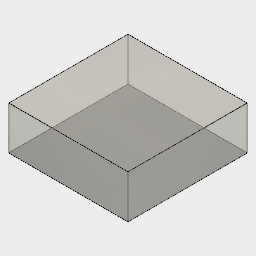
Poseidon thrust frame motor mount blocks (Autodesk Fusion 360 design; units mm, degrees)
Autodesk Fusion 360 part; units mm, degrees
sketch "Sketch1" plane through (0, 0, 0) normal (0, 1, 0) x (1, 0, 0)
  line L0 (0, 0) -> (34.925, 0)
  line L1 (34.925, 0) -> (34.925, 34.925)
  line L2 (34.925, 34.925) -> (0, 34.925)
  line L3 (0, 34.925) -> (0, 0)
  line L4 (0, 0) -> (34.925, 0)
  line L5 (34.925, 0) -> (34.925, 34.925)
  dimension "d1" = 34.925
  dimension "d2" = 34.925
  measures "d1" distance of L0.start L0.end
  measures "d2" distance of L0.end L1.end
extrude "Extrude1" add sketch "Sketch1" along normal blind 12.7
